y_belt_holder (Autodesk Fusion 360 design; units mm, degrees)
Autodesk Fusion 360 part; units mm, degrees
sketch "Sketch1" plane through (0, 0, 0) normal (0, 0, 1) x (1, 0, 0)
  circle A0 centre (0, 0) radius 3.5
  circle A1 centre (12, 0) radius 3.5
  line L0 (-12, 10.5) -> (-2, 10.5)
  line L1 (-2, 10.5) -> (-2, 5.5)
  line L2 (-2, 5.5) -> (-12, 5.5)
  line L3 (-12, 5.5) -> (-12, 10.5)
  line L4 (14, 5.5) -> (24, 5.5)
  line L5 (24, 5.5) -> (24, 10.5)
  line L6 (24, 10.5) -> (14, 10.5)
  line L7 (14, 10.5) -> (14, 5.5)
  line L8 (-12, 3.3) -> (-10, 3.3)
  line L9 (-7, 0.3) -> (-7, -4.5)
  line L10 (-7, -4.5) -> (-12, -4.5)
  line L11 (-12, -4.5) -> (-12, 3.3)
  line L12 (22, 3.3) -> (24, 3.3)
  line L13 (24, 3.3) -> (24, -4.5)
  line L14 (24, -4.5) -> (19, -4.5)
  line L15 (19, -4.5) -> (19, 0.3)
  arc A2 (-7, 0.3) -> (-10, 3.3) centre (-10, 0.3) ccw
  arc A3 (22, 3.3) -> (19, 0.3) centre (22, 0.3) ccw
  dimension "d1" = 7
  dimension "d2" = 12
  dimension "d3" = 2
  dimension "d4" = 5.5
  dimension "d5" = 2
  dimension "d6" = 2.2
  dimension "d7" = 5
  dimension "d9" = 15
  dimension "d10" = 12
  dimension "d11" = 5
  dimension "d12" = 5
  dimension "d13" = 3
  constraint coincident A0.centre origin
  constraint equal A0 A1
  constraint horizontal A0.centre A1.centre
  constraint horizontal L0
  constraint vertical L1
  constraint horizontal L2
  constraint vertical L3
  constraint horizontal L4
  constraint vertical L5
  constraint horizontal L6
  constraint vertical L7
  constraint horizontal L1.end L4.start
  constraint horizontal L0.end L6.end
  constraint equal L0 L6
  constraint horizontal L8
  constraint vertical L9
  constraint horizontal L10
  constraint vertical L11
  constraint horizontal L12
  constraint vertical L13
  constraint horizontal L14
  constraint vertical L15
  constraint horizontal L9.end L14.end
  constraint vertical L2.end L8.start
  constraint vertical L4.end L12.end
  constraint tangent L8 A2
  constraint tangent L9 A2
  constraint tangent L12 A3
  constraint tangent L15 A3
  constraint equal A2 A3
  constraint horizontal L8.start L12.end
  measures "d1" diameter of A0
  measures "d2" distance of A0.centre A1.centre
  measures "d3" distance of A0.centre L1
  measures "d4" distance of A0.centre L2
  measures "d5" distance of A1.centre L7
  measures "d6" distance of L4 L12
  measures "d7" distance of L1 L9
  measures "d9" distance of L6 L14
  measures "d10" distance of A0.centre L11
  measures "d11" distance of L7 L15
  measures "d12" distance of L0.start L2.end
  measures "d13" radius of A2
extrude "Extrude1" add sketch "Sketch1" along normal blind 7 makes body 1 at (24, 0.7, 2.3333) makes body 2 at (-8.6667, 10.5, 2.3333) makes body 3 at (3.4826, -0.3485, 4.6667) makes body 4 at (15.4826, -0.3485, 4.6667) makes body 5 at (20.6667, 10.5, 2.3333) makes body 6 at (-12, -1.9, 2.3333)
sketch "Sketch2" plane through (0, 0, 0) normal (0, 0, 1) x (1, 0, 0)
  line L0 (24, 10.5) -> (-12, 10.5)
  line L1 (-12, 10.5) -> (-12, -4.5)
  line L2 (-12, -4.5) -> (24, -4.5)
  line L3 (24, -4.5) -> (24, 10.5)
  point P0 (24, 10.5)
  point P1 (-12, -4.5)
  constraint horizontal L0
  constraint vertical L1
  constraint horizontal L2
  constraint vertical L3
  constraint coincident P1 L1.end
  constraint coincident P0 L0.start
extrude "Extrude2" add sketch "Sketch2" against normal blind 3 bodies 1 2 3 4 5 6
sketch "Sketch3" plane through (0, 0, -3) normal (0, 0, -1) x (-1, 0, 0)
  line L0 (-24, 10.5) -> (-24, -4.5)
  line L1 (-24, -4.5) -> (12, -4.5)
  line L2 (12, -4.5) -> (12, 10.5)
  line L3 (12, 10.5) -> (-24, 10.5)
  line L4 (12, 10.5) -> (12, 15.5)
  line L5 (12, 15.5) -> (-8.6, 29.85)
  line L6 (-8.6, 29.85) -> (-13.6, 29.85)
  line L7 (-13.6, 29.85) -> (-13.6, 28.35)
  line L8 (-13.6, 28.35) -> (-24, 28.35)
  line L9 (-24, 28.35) -> (-24, 10.5)
  line L10 (-14, 5.5) -> (-24, 5.5)
  dimension "d18" = 22.85
  dimension "d19" = 5
  dimension "d20" = 1.5
  dimension "d21" = 10.4
  dimension "d22" = 5
  constraint coincident L2.end L3.start
  constraint perpendicular L3 L4
  constraint perpendicular L4 L6
  constraint perpendicular L6 L7
  constraint perpendicular L7 L8
  constraint coincident L0.start L3.end
  constraint vertical L9
  measures "d18" distance of L8 L10
  measures "d19" distance of L2.end L4.end
  measures "d20" distance of L6 L8
  measures "d21" distance of L7 L9
  measures "d22" distance of L5.end L6.end
extrude "Extrude3" add sketch "Sketch3" against normal blind 16 contours L3 L4 L5 L6 L7 L8 L9 bodies 1
extrude "Extrude4" add 1 faces at (8.5333, 13.1167, -3) along direction (0, 0, -1) blind 4 on bodies 1 bodies 1
sketch "Sketch4" plane through (0, 28.35, 0) normal (0, 1, 0) x (-1, 0, 0)
  line L0 (-13.6, -7) -> (-13.6, 13)
  line L1 (-13.6, 13) -> (-24, 13)
  line L2 (-24, 13) -> (-24, -7)
  line L3 (-24, -7) -> (-13.6, -7)
  circle A0 centre (-19, -3) radius 1.6
  circle A1 centre (-19, 9) radius 1.6
  point P0 (-24, 3)
  dimension "d27" = 3.2
  dimension "d28" = 12
  dimension "d29" = 6
  dimension "d30" = 5.4
  constraint equal A0 A1
  constraint midpoint L2 P0
  constraint vertical A0.centre A1.centre
  measures "d27" diameter of A0
  measures "d28" distance of A0.centre A1.centre
  measures "d29" vertical distance of A0.centre P0
  measures "d30" distance of L0 A0.centre
extrude "Extrude5" cut sketch "Sketch4" against normal through all contours A0 | A1 bodies 1
sketch "Sketch5" plane through (0, -4.5, 0) normal (0, -1, 0) x (1, 0, 0)
  line L0 (19, 7) -> (19, 0)
  line L1 (19, 0) -> (-7, 0)
  line L2 (-7, 0) -> (-7, 7)
  line L3 (24, 7) -> (19, 7)
  line L4 (-12, 7) -> (-12, -7)
  line L5 (-12, -7) -> (24, -7)
  line L6 (24, -7) -> (24, 7)
  circle A0 centre (19, -3) radius 1.6
  circle A1 centre (19, -3) radius 1.6
  circle A2 centre (19, 9) radius 3.1
  circle A3 centre (19, -3) radius 3.1
  circle A4 centre (19, 9) radius 1.6
  line L7 (15.9, -3) -> (15.9, 0)
  line L8 (15.9, 0) -> (18.219, 0)
  line L9 (19, 3.2) -> (21.6847, -1.45)
  line L10 (-7, 7) -> (-12, 7)
  dimension "d32" = 6.2
  dimension "d39" = 30
  constraint concentric A0 A3
  constraint equal A2 A3
  constraint coincident A2.centre A4.centre
  constraint coincident A3 L7.start
  constraint coincident L1 L7.end
  constraint perpendicular L1 L7
  constraint coincident A3 L8.end
  constraint coincident L1 L8.end
  constraint coincident L0 L9.start
  constraint coincident A3 L9.end
  constraint tangent A3 L9
  constraint horizontal A0.centre L7.start
  measures "d32" diameter of A2
  measures "d39" angle of L0 L9
extrude "Extrude6" cut sketch "Sketch5" against normal blind 18 contours L0 L3 A2 | L0 L3 A2 | A4 bodies 1
chamfer "Chamfer1" distance 1.5 angle 45 4 edges at (-2, 5.5, 3.5) (14, 5.5, 3.5) (-7, -4.5, 3.5) (19, -4.5, 2.95) on bodies 1
chamfer "Chamfer2" distance 0.7 angle 45 15 edges at (-7.75, 5.5, 7) (-2.75, 6.25, 7) (-2, 8.75, 7) (-7, -1.35, 7) (-7.8787, 2.4213, 7) (-11, 3.3, 7) (-10.25, -4.5, 7) (-7.75, -3.75, 7) (-3.2631, -1.2657, 7) (8.7369, -1.2657, 7) (14, 8.75, 7) (14.75, 6.25, 7) (22.6843, 5.5, 7) (22.6843, -4.5, 7) (23, 3.3, 7) on bodies 1
chamfer "Chamfer4" distance 2 angle 45 10 edges at (-12, 5.5, -7) (-1.7, 22.675, -7) (11.1, 29.85, -7) (24, 11.925, -7) (6, -4.5, -7) (6, 10.5, 13) (-12, 13, 13) (-1.7, 22.675, 13) (11.1, 29.85, 13) (24, 19.425, 13) on bodies 1
extrude "Extrude7" cut sketch "Sketch5" against normal blind 3 contours L0 A3 L9 | L0 L1 A3 | L1 A3 L7 L8 picked at (18.621, -0.48) bodies 1
equation "d5 = d3"
equation "d11 = d7"
equation "d23 = -6 mm - 10 mm"
equation "d29 = d28 / 2"
